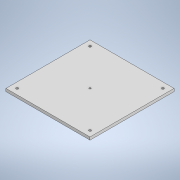
# Autodesk Inventor part: Plate
Saved by Autodesk Inventor 2020.3 (Build 243373000, 373)
## iProperties
Created: 2020-10-30
Part Number: Plate
Material: Generic
Document SubType Name: Modeling
Designer: Naude Conradie
Density: 1 g/cm^3
Appearance: Default
Author: Naude Conradie
Autodesk Inventor part; units mm, degrees
ref_plane "YZ Plane" through (0, 0, 0) normal (1, 0, 0) x (0, 1, 0)
ref_plane "XZ Plane" through (0, 0, 0) normal (0, 1, 0) x (-1, 0, 0)
ref_plane "XY Plane" through (0, 0, 0) normal (0, 0, 1) x (1, 0, 0)
sketch "Sketch1" plane through (0, 0, 0) normal (0, 1, 0) x (-1, 0, 0)
  line L0 (0, 0) -> (300, 0)
  line L1 (300, 0) -> (300, -300)
  line L2 (300, -300) -> (0, -300)
  line L3 (0, -300) -> (0, 0)
  dimension "d0" = 300
  dimension "d1" = 300
  constraints: 8 end point, 2 parallel, 1 horizontal, 1 perpendicular
  measures "d0" distance of L1.end L2.end
  measures "d1" distance of L0.end L1.end
extrude "Extrusion1" add sketch "Sketch1" along normal blind 10
sketch "Sketch2" plane through (0, 10, 0) normal (0, 1, 0) x (1, 0, 0)
  line L0 (-300, 0) -> (0, 0) projected
  line L1 (0, 0) -> (0, 300) projected
  point P0 (-20, 20)
  point P1 (-20, 280)
  point P2 (-280, 20)
  point P3 (-280, 280)
  dimension "d4" = 20
  dimension "d5" = 20
  dimension "d8" = 260
  dimension "d11" = 260
  constraints: 1 horizontal, 1 vertical, 3 other
  measures "d4" horizontal distance of L0.end point (-20, 20)
  measures "d5" horizontal distance of L0.end point (-20, 20)
  measures "d8" distance of point (-20, 20) point (-20, 280)
  measures "d11" distance of point (-20, 20) point (-280, 20)
hole "Hole1" at (-20, 10, -20) at (-20, 10, -280) at (-280, 10, -20) at (-280, 10, -280) direction (0, -1, 0) diameter 8 end through all
sketch "Sketch3" plane through (0, 10, 0) normal (0, 1, 0) x (1, 0, 0)
  line L0 (-300, 300) -> (-300, 0) projected
  line L1 (0, 300) -> (-300, 300) projected
  point P0 (0, 0)
  point P1 (-150, 150)
  dimension "d21" = 150
  dimension "d22" = 150
  measures "d21" horizontal distance of point (0, 0) point (-150, 150)
  measures "d22" horizontal distance of point (0, 0) point (-150, 150)
hole "Hole2" at (-150, 10, -150) direction (0, -1, 0) diameter 6 end through all
body "Solid1"
